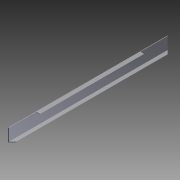
# Autodesk Inventor part: frame U 1 by 3 long
Saved by Autodesk Inventor 2012 (Build 160160000, 160)
## iProperties
Created: 2013-07-20
Part Number: frame U 1 by 3 long
Material: Default
Document SubType Name: Modeling
Designer: Bryce
Density: 1 g/cm^3
Author: Bryce
Autodesk Inventor part; units mm, degrees
ref_plane "YZ Plane" through (0, 0, 0) normal (1, 0, 0) x (0, 1, 0)
ref_plane "XZ Plane" through (0, 0, 0) normal (0, 1, 0) x (-1, 0, 0)
ref_plane "XY Plane" through (0, 0, 0) normal (0, 0, 1) x (1, 0, 0)
sketch "Sketch1" plane through (0, 0, 0) normal (0, 0, 1) x (1, 0, 0)
  line L0 (0, 0) -> (25.4, 0)
  line L1 (25.4, 76.2) -> (0, 76.2)
  line L2 (0, 76.2) -> (0, 0)
  line L3 (25.4, 3.175) -> (3.175, 3.175)
  line L4 (3.175, 3.175) -> (3.175, 73.025)
  line L5 (3.175, 73.025) -> (25.4, 73.025)
  line L6 (25.4, 0) -> (25.4, 3.175)
  line L7 (25.4, 73.025) -> (25.4, 76.2)
  dimension "d0" = 76.2
  dimension "d1" = 25.4
  dimension "d2" = 3.175
  dimension "d3" = 3.175
  dimension "d4" = 3.175
  constraints: 16 end point, 4 parallel, 3 perpendicular, 2 horizontal, 1 collinear
  measures "d0" distance of L1.end L0.start
  measures "d1" distance of L0.start L0.end
  measures "d2" distance between parallel lines of L0 L3
  measures "d3" distance between parallel lines of L4 L2
  measures "d4" distance between parallel lines of L1 L5
extrude "Extrusion1" add sketch "Sketch1" along normal blind 965.2
sketch "Sketch2" plane through (0, 76.2, 0) normal (0, 1, 0) x (1, 0, 0)
  line L0 (0, -965.2) -> (25.4, -965.2) projected
  line L1 (25.4, 0) -> (25.4, -965.2) projected
  line L2 (25.4, 0) -> (0, 0) projected
  line L3 (0, 0) -> (0, -965.2) projected
  line L4 (0, -965.2) -> (25.4, -939.8)
  line L5 (0, 0) -> (25.4, -25.4)
  line L6 (3.175, -962.025) -> (3.175, -796.925)
  line L7 (3.175, -796.925) -> (25.4, -796.925)
  line L8 (3.175, -3.175) -> (3.175, -168.275)
  line L9 (3.175, -168.275) -> (25.4, -168.275)
  dimension "d7" = 45
  dimension "d8" = 3.175
  dimension "d9" = 165.1
  dimension "d10" = 165.1
  constraints: 12 end point, 6 point on line, 3 perpendicular, 2 parallel, 1 collinear
  measures "d7" angle of L0 L4
  measures "d8" distance between parallel lines of L6 L3
  measures "d9" distance of L6.start L6.end
  measures "d10" distance of L8.start L8.end
extrude "Extrusion2" cut sketch "Sketch2" against normal through all contours L4 L1 L0 | L2 L1 L5
extrude "Extrusion3" cut sketch "Sketch2" against normal up to next contours L6 L7 L1 L4 | L5 L1 L9 L8
equation "\"d3\" = d2"
equation "\"d4\" = d2"
equation "\"d10\" = d9"
body "Solid1"
